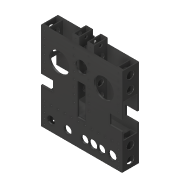
# Autodesk Inventor part: Kermit Elbow
Saved by Autodesk Inventor 2018.2 (Build 222227000, 227)
## iProperties
Created: 2018-02-12
Part Number: Kermit Elbow
Material: Glass
Document SubType Name: Modeling
Designer: lopez.xavier
Density: 2.18 g/cm^3
Appearance: Dark Gray
Author: lopez.xavier
Autodesk Inventor part; units mm, degrees
ref_plane "YZ Plane" through (0, 0, 0) normal (1, 0, 0) x (0, 1, 0)
ref_plane "XZ Plane" through (0, 0, 0) normal (0, 1, 0) x (-1, 0, 0)
ref_plane "XY Plane" through (0, 0, 0) normal (0, 0, 1) x (1, 0, 0)
sketch "Sketch1" plane through (0, 0, 0) normal (0, 0, 1) x (1, 0, 0)
  line L0 (0, 0) -> (304.8, 0)
  line L1 (304.8, 0) -> (304.8, 330.2)
  line L2 (304.8, 330.2) -> (0, 330.2)
  line L3 (0, 330.2) -> (0, 0)
  line L4 (0, 171.45) -> (45.72, 171.45)
  line L5 (45.72, 171.45) -> (45.72, 133.35)
  line L6 (45.72, 133.35) -> (0, 133.35)
  line L7 (0, 133.35) -> (0, 171.45)
  line L8 (304.8, 171.45) -> (259.08, 171.45)
  line L9 (259.08, 171.45) -> (259.08, 133.35)
  line L10 (259.08, 133.35) -> (304.8, 133.35)
  line L11 (304.8, 133.35) -> (304.8, 171.45)
  circle A0 centre (12.7, 317.5) radius 2.54
  circle A1 centre (292.1, 317.5) radius 2.54
  circle A2 centre (12.7, 292.1) radius 2.54
  circle A3 centre (12.7, 266.7) radius 2.54
  circle A4 centre (12.7, 241.3) radius 2.54
  circle A5 centre (12.7, 215.9) radius 2.54
  circle A6 centre (12.7, 190.5) radius 2.54
  circle A7 centre (292.1, 292.1) radius 2.54
  circle A8 centre (292.1, 266.7) radius 2.54
  circle A9 centre (292.1, 241.3) radius 2.54
  circle A10 centre (292.1, 215.9) radius 2.54
  circle A11 centre (292.1, 190.5) radius 2.54
  dimension "d0" = 304.8
  dimension "d1" = 330.2
  dimension "d2" = 158.75
  dimension "d3" = 38.1
  dimension "d4" = 45.72
  dimension "d5" = 45.72
  dimension "d6" = 5.08
  dimension "d7" = 5.08
  dimension "d8" = 12.7
  dimension "d9" = 12.7
  dimension "d10" = 12.7
  dimension "d11" = 12.7
  dimension "d14" = 25.4
  dimension "d21" = 25.4
  constraints: 24 end point, 12 centre point, 6 parallel, 4 point on line, 3 horizontal, 3 perpendicular, 2 vertical, 20 other
  measures "d0" distance of L0.start L0.end
  measures "d1" distance of L2.end L0.start
  measures "d2" distance between parallel lines of L2 L8
  measures "d3" distance between parallel lines of L4 L6
  measures "d4" distance between parallel lines of L3 L5
  measures "d5" distance between parallel lines of L1 L9
  measures "d6" diameter of A0
  measures "d7" diameter of A1
  measures "d8" distance from line of L2 A1.centre
  measures "d9" distance from line of L1 A1.centre
  measures "d10" distance from line of L2 A0.centre
  measures "d11" distance from line of L3 A0.centre
  measures "d14" distance of A0.centre A2.centre
  measures "d21" distance of A1.centre A7.centre
sketch "Sketch1 outline for Extrusion1" plane through (0, 0, 0) normal (0, 0, 1) x (1, 0, 0)
  line L0 (0, 330.2) -> (0, 171.45)
  line L1 (304.8, 330.2) -> (0, 330.2)
  line L2 (304.8, 171.45) -> (304.8, 330.2)
  line L3 (304.8, 171.45) -> (259.08, 171.45)
  line L4 (259.08, 171.45) -> (259.08, 133.35)
  line L5 (259.08, 133.35) -> (304.8, 133.35)
  line L6 (304.8, 0) -> (304.8, 133.35)
  line L7 (0, 0) -> (304.8, 0)
  line L8 (0, 133.35) -> (0, 0)
  line L9 (0, 133.35) -> (45.72, 133.35)
  line L10 (45.72, 133.35) -> (45.72, 171.45)
  line L11 (45.72, 171.45) -> (0, 171.45)
  circle A0 centre (12.7, 190.5) radius 2.54
  circle A1 centre (12.7, 215.9) radius 2.54
  circle A2 centre (12.7, 241.3) radius 2.54
  circle A3 centre (292.1, 190.5) radius 2.54
  circle A4 centre (292.1, 215.9) radius 2.54
  circle A5 centre (292.1, 241.3) radius 2.54
  circle A6 centre (12.7, 266.7) radius 2.54
  circle A7 centre (12.7, 292.1) radius 2.54
  circle A8 centre (12.7, 317.5) radius 2.54
  circle A9 centre (292.1, 266.7) radius 2.54
  circle A10 centre (292.1, 292.1) radius 2.54
  circle A11 centre (292.1, 317.5) radius 2.54
extrude "Extrusion1" add sketch "Sketch1 outline for Extrusion1" along normal blind 63.5
sketch "Sketch2" plane through (304.8, 171.45, 0) normal (1, 0, 0) x (0, 0, -1)
  line L0 (0, 158.75) -> (-63.5, 158.75) projected
  line L1 (0, -171.45) -> (-63.5, -171.45) projected
  line L2 (-57.531, 158.75) -> (-5.969, 158.75)
  line L3 (-5.969, 158.75) -> (-5.969, -171.45)
  line L4 (-5.969, -171.45) -> (-57.531, -171.45)
  line L5 (-57.531, -171.45) -> (-57.531, 158.75)
  line L6 (0, 0) -> (0, 158.75) projected
  line L7 (-63.5, 0) -> (-63.5, 158.75) projected
  dimension "d28" = 5.969
  dimension "d29" = 5.969
  constraints: 8 end point, 2 parallel, 2 point on line, 1 horizontal, 1 perpendicular
  measures "d28" distance between parallel lines of L6 L3
  measures "d29" distance between parallel lines of L7 L5
sketch "Sketch2 outline for Extrusion2" plane through (304.8, 171.45, 0) normal (1, 0, 0) x (0, 0, -1)
  line L0 (-57.531, 158.75) -> (-5.969, 158.75)
  line L1 (-5.969, 158.75) -> (-5.969, -171.45)
  line L2 (-5.969, -171.45) -> (-57.531, -171.45)
  line L3 (-57.531, -171.45) -> (-57.531, 158.75)
extrude "Extrusion2" cut sketch "Sketch2 outline for Extrusion2" against normal blind 508
sketch "Sketch3" plane through (0, 0, 63.5) normal (0, 0, 1) x (1, 0, 0)
  circle A0 centre (124.46, 317.5) radius 2.54
  line L0 (304.8, 330.2) -> (0, 330.2) projected
  line L1 (0, 330.2) -> (0, 171.45) projected
  circle A1 centre (124.46, 292.1) radius 2.54
  circle A2 centre (124.46, 266.7) radius 2.54
  circle A3 centre (124.46, 241.3) radius 2.54
  circle A4 centre (124.46, 215.9) radius 2.54
  circle A5 centre (124.46, 190.5) radius 2.54
  circle A6 centre (124.46, 165.1) radius 2.54
  circle A7 centre (124.46, 139.7) radius 2.54
  circle A8 centre (180.34, 317.5) radius 2.54
  circle A9 centre (180.34, 292.1) radius 2.54
  circle A10 centre (180.34, 266.7) radius 2.54
  circle A11 centre (180.34, 241.3) radius 2.54
  circle A12 centre (180.34, 215.9) radius 2.54
  circle A13 centre (180.34, 190.5) radius 2.54
  circle A14 centre (180.34, 165.1) radius 2.54
  circle A15 centre (180.34, 139.7) radius 2.54
  point P0 (0, 0)
  dimension "d32" = 5.08
  dimension "d33" = 12.7
  dimension "d34" = 124.46
  dimension "d37" = 25.4
  dimension "d40" = 55.88
  constraints: 16 centre point, 1 horizontal, 1 vertical, 30 other
  measures "d32" diameter of A0
  measures "d33" distance from line of L0 A0.centre
  measures "d34" distance from line of L1 A0.centre
  measures "d37" distance of A0.centre A1.centre
  measures "d40" distance of A0.centre A8.centre
sketch "Sketch3 outline for Extrusion3" plane through (0, 0, 63.5) normal (0, 0, 1) x (1, 0, 0)
  circle A0 centre (124.46, 317.5) radius 2.54
  circle A1 centre (124.46, 292.1) radius 2.54
  circle A2 centre (124.46, 266.7) radius 2.54
  circle A3 centre (124.46, 241.3) radius 2.54
  circle A4 centre (124.46, 215.9) radius 2.54
  circle A5 centre (124.46, 190.5) radius 2.54
  circle A6 centre (124.46, 165.1) radius 2.54
  circle A7 centre (124.46, 139.7) radius 2.54
  circle A8 centre (180.34, 317.5) radius 2.54
  circle A9 centre (180.34, 292.1) radius 2.54
  circle A10 centre (180.34, 266.7) radius 2.54
  circle A11 centre (180.34, 241.3) radius 2.54
  circle A12 centre (180.34, 215.9) radius 2.54
  circle A13 centre (180.34, 190.5) radius 2.54
  circle A14 centre (180.34, 165.1) radius 2.54
  circle A15 centre (180.34, 139.7) radius 2.54
extrude "Extrusion3" cut sketch "Sketch3 outline for Extrusion3" against normal blind 508
sketch "Sketch4" plane through (0, 0, 63.5) normal (0, 0, 1) x (1, 0, 0)
  line L0 (137.16, 216.662) -> (167.64, 216.662)
  line L1 (167.64, 216.662) -> (167.64, 97.282)
  line L2 (167.64, 97.282) -> (137.16, 97.282)
  line L3 (137.16, 97.282) -> (137.16, 216.662)
  circle A0 centre (124.46, 215.9) radius 2.54 projected
  line L4 (304.8, 330.2) -> (0, 330.2) projected
  point P0 (0, 0)
  dimension "d45" = 30.48
  dimension "d46" = 12.7
  dimension "d47" = 113.538
  dimension "d48" = 119.38
  constraints: 8 end point, 2 parallel, 1 horizontal, 1 perpendicular
  measures "d45" distance between parallel lines of L3 L1
  measures "d46" distance from line of A0.centre L3
  measures "d47" distance between parallel lines of L4 L0
  measures "d48" distance between parallel lines of L0 L2
sketch "Sketch4 outline for Extrusion4" plane through (0, 0, 63.5) normal (0, 0, 1) x (1, 0, 0)
  line L0 (137.16, 216.662) -> (167.64, 216.662)
  line L1 (167.64, 216.662) -> (167.64, 97.282)
  line L2 (167.64, 97.282) -> (137.16, 97.282)
  line L3 (137.16, 97.282) -> (137.16, 216.662)
extrude "Extrusion4" cut sketch "Sketch4 outline for Extrusion4" against normal blind 508
sketch "Sketch5" plane through (304.8, 171.45, 57.531) normal (0, 0, -1) x (-1, 0, 0)
  line L0 (304.8, 0) -> (304.8, 158.75) projected
  line L1 (304.8, 158.75) -> (279.4, 158.75)
  line L2 (279.4, 158.75) -> (279.4, 57.15)
  line L3 (279.4, 57.15) -> (304.8, 57.15)
  line L4 (304.8, 57.15) -> (304.8, 158.75)
  line L5 (0, 158.75) -> (0, 0) projected
  line L6 (0, 158.75) -> (25.4, 158.75)
  line L7 (25.4, 158.75) -> (25.4, 57.15)
  line L8 (25.4, 57.15) -> (0, 57.15)
  line L9 (0, 57.15) -> (0, 158.75)
  point P0 (304.8, -171.45)
  dimension "d51" = 25.4
  dimension "d52" = 101.6
  dimension "d53" = 25.4
  dimension "d54" = 101.6
  constraints: 16 end point, 4 parallel, 2 horizontal, 2 perpendicular
  measures "d51" distance of L3.end L2.end
  measures "d52" distance of L2.end L1.end
  measures "d53" distance of L7.end L8.end
  measures "d54" distance of L6.end L7.end
sketch "Sketch5 outline for Extrusion5" plane through (304.8, 171.45, 57.531) normal (0, 0, -1) x (-1, 0, 0)
  line L0 (304.8, 57.15) -> (304.8, 158.75)
  line L1 (279.4, 57.15) -> (304.8, 57.15)
  line L2 (279.4, 158.75) -> (279.4, 57.15)
  line L3 (304.8, 158.75) -> (279.4, 158.75)
  line L4 (0, 158.75) -> (25.4, 158.75)
  line L5 (25.4, 158.75) -> (25.4, 57.15)
  line L6 (25.4, 57.15) -> (0, 57.15)
  line L7 (0, 57.15) -> (0, 158.75)
extrude "Extrusion5" add sketch "Sketch5 outline for Extrusion5" along normal blind 51.562
sketch "Sketch6" plane through (0, 0, 63.5) normal (0, 0, 1) x (1, 0, 0)
  circle A0 centre (292.1, 241.3) radius 2.54 projected
  circle A1 centre (292.1, 266.7) radius 2.54 projected
  circle A2 centre (292.1, 292.1) radius 2.54 projected
  circle A3 centre (292.1, 317.5) radius 2.54 projected
  circle A4 centre (12.7, 317.5) radius 2.54 projected
  circle A5 centre (12.7, 292.1) radius 2.54 projected
  circle A6 centre (12.7, 266.7) radius 2.54 projected
  circle A7 centre (12.7, 241.3) radius 2.54 projected
  point P0 (0, 0)
sketch "Sketch6 outline for Extrusion6" plane through (0, 0, 63.5) normal (0, 0, 1) x (1, 0, 0)
  circle A0 centre (292.1, 241.3) radius 2.54
  circle A1 centre (292.1, 266.7) radius 2.54
  circle A2 centre (292.1, 292.1) radius 2.54
  circle A3 centre (292.1, 317.5) radius 2.54
  circle A4 centre (12.7, 317.5) radius 2.54
  circle A5 centre (12.7, 292.1) radius 2.54
  circle A6 centre (12.7, 266.7) radius 2.54
  circle A7 centre (12.7, 241.3) radius 2.54
extrude "Extrusion6" cut sketch "Sketch6 outline for Extrusion6" against normal blind 63.5
sketch "Sketch7" plane through (0, 0, 63.5) normal (0, 0, 1) x (1, 0, 0)
  circle A0 centre (68.58, 241.3) radius 38.1
  circle A1 centre (236.22, 241.3) radius 38.1
  circle A2 centre (12.7, 266.7) radius 2.54 projected
  circle A3 centre (292.1, 241.3) radius 2.54 projected
  line L0 (304.8, 330.2) -> (0, 330.2) projected
  point P0 (0, 0)
  dimension "d59" = 76.2
  dimension "d60" = 76.2
  dimension "d61" = 55.88
  dimension "d62" = 55.88
  dimension "d63" = 88.9
  dimension "d64" = 88.9
  constraints: 2 centre point
  measures "d59" diameter of A0
  measures "d60" diameter of A1
  measures "d61" horizontal distance of A2.centre A0.centre
  measures "d62" distance of A3.centre A1.centre
  measures "d63" distance from line of L0 A0.centre
  measures "d64" distance from line of L0 A1.centre
sketch "Sketch7 outline for Extrusion7" plane through (0, 0, 63.5) normal (0, 0, 1) x (1, 0, 0)
  circle A0 centre (68.58, 241.3) radius 38.1
  circle A1 centre (236.22, 241.3) radius 38.1
extrude "Extrusion7" cut sketch "Sketch7 outline for Extrusion7" against normal blind 63.5
sketch "Sketch8" plane through (304.8, 0, 57.531) normal (0, 0, -1) x (-1, 0, 0)
  line L0 (111.76, 152.4) -> (137.16, 152.4)
  line L1 (137.16, 152.4) -> (137.16, 355.6)
  line L2 (137.16, 355.6) -> (111.76, 355.6)
  line L3 (111.76, 355.6) -> (111.76, 152.4)
  line L4 (0, 330.2) -> (304.8, 330.2) projected
  circle A0 centre (124.46, 241.3) radius 2.54 projected
  line L5 (193.04, 152.4) -> (167.64, 152.4)
  line L6 (167.64, 152.4) -> (167.64, 355.6)
  line L7 (167.64, 355.6) -> (193.04, 355.6)
  line L8 (193.04, 355.6) -> (193.04, 152.4)
  circle A1 centre (180.34, 241.3) radius 2.54 projected
  point P0 (304.8, 0)
  dimension "d67" = 25.4
  dimension "d68" = 203.2
  dimension "d69" = 25.4
  dimension "d70" = 12.7
  dimension "d71" = 203.2
  dimension "d72" = 25.4
  dimension "d73" = 25.4
  dimension "d74" = 12.7
  constraints: 16 end point, 4 parallel, 2 horizontal, 2 perpendicular
  measures "d67" distance of L2.end L1.end
  measures "d68" distance of L1.end L0.end
  measures "d69" distance between parallel lines of L4 L2
  measures "d70" distance from line of A0.centre L3
  measures "d71" distance between parallel lines of L7 L5
  measures "d72" distance between parallel lines of L6 L8
  measures "d73" distance between parallel lines of L4 L7
  measures "d74" distance from line of A1.centre L8
sketch "Sketch8 outline for Extrusion8" plane through (304.8, 0, 57.531) normal (0, 0, -1) x (-1, 0, 0)
  line L0 (111.76, 355.6) -> (111.76, 152.4)
  line L1 (137.16, 355.6) -> (111.76, 355.6)
  line L2 (111.76, 152.4) -> (137.16, 152.4)
  line L3 (137.16, 152.4) -> (137.16, 355.6)
  circle A0 centre (124.46, 241.3) radius 2.54
  line L4 (193.04, 152.4) -> (167.64, 152.4)
  line L5 (193.04, 355.6) -> (193.04, 152.4)
  line L6 (167.64, 152.4) -> (167.64, 355.6)
  line L7 (167.64, 355.6) -> (193.04, 355.6)
  circle A1 centre (180.34, 241.3) radius 2.54
extrude "Extrusion8" add sketch "Sketch8 outline for Extrusion8" along normal blind 51.562
sketch "Sketch9" plane through (0, 0, 0) normal (0, 0, -1) x (-1, 0, 0)
  circle A0 centre (-180.34, 342.9) radius 2.54
  line L0 (-193.04, 355.6) -> (-193.04, 330.2) projected
  line L1 (-167.64, 355.6) -> (-193.04, 355.6) projected
  circle A1 centre (-180.34, 317.5) radius 2.54
  circle A2 centre (-180.34, 292.1) radius 2.54
  circle A3 centre (-180.34, 266.7) radius 2.54
  circle A4 centre (-180.34, 241.3) radius 2.54
  circle A5 centre (-180.34, 215.9) radius 2.54
  circle A6 centre (-180.34, 190.5) radius 2.54
  circle A7 centre (-180.34, 165.1) radius 2.54
  circle A8 centre (-124.46, 342.9) radius 2.54
  circle A9 centre (-124.46, 317.5) radius 2.54
  circle A10 centre (-124.46, 292.1) radius 2.54
  circle A11 centre (-124.46, 266.7) radius 2.54
  circle A12 centre (-124.46, 241.3) radius 2.54
  circle A13 centre (-124.46, 215.9) radius 2.54
  circle A14 centre (-124.46, 190.5) radius 2.54
  circle A15 centre (-124.46, 165.1) radius 2.54
  point P0 (0, 0)
  dimension "d77" = 5.08
  dimension "d78" = 12.7
  dimension "d79" = 12.7
  dimension "d82" = 25.4
  dimension "d85" = 55.88
  constraints: 16 centre point, 1 horizontal, 1 vertical, 30 other
  measures "d77" diameter of A0
  measures "d78" distance from line of L0 A0.centre
  measures "d79" distance from line of L1 A0.centre
  measures "d82" distance of A0.centre A1.centre
  measures "d85" distance of A0.centre A8.centre
sketch "Sketch9 outline for Extrusion9" plane through (0, 0, 0) normal (0, 0, -1) x (-1, 0, 0)
  circle A0 centre (-180.34, 342.9) radius 2.54
  circle A1 centre (-180.34, 317.5) radius 2.54
  circle A2 centre (-180.34, 292.1) radius 2.54
  circle A3 centre (-180.34, 266.7) radius 2.54
  circle A4 centre (-180.34, 241.3) radius 2.54
  circle A5 centre (-180.34, 215.9) radius 2.54
  circle A6 centre (-180.34, 190.5) radius 2.54
  circle A7 centre (-180.34, 165.1) radius 2.54
  circle A8 centre (-124.46, 342.9) radius 2.54
  circle A9 centre (-124.46, 317.5) radius 2.54
  circle A10 centre (-124.46, 292.1) radius 2.54
  circle A11 centre (-124.46, 266.7) radius 2.54
  circle A12 centre (-124.46, 241.3) radius 2.54
  circle A13 centre (-124.46, 215.9) radius 2.54
  circle A14 centre (-124.46, 190.5) radius 2.54
  circle A15 centre (-124.46, 165.1) radius 2.54
extrude "Extrusion9" cut sketch "Sketch9 outline for Extrusion9" against normal blind 63.5
sketch "Sketch10" plane through (304.8, 0, 57.531) normal (0, 0, -1) x (-1, 0, 0)
  line L0 (304.8, 0) -> (0, 0) projected
  line L1 (0, 0) -> (25.4, 0)
  line L2 (25.4, 0) -> (25.4, 101.6)
  line L3 (25.4, 101.6) -> (0, 101.6)
  line L4 (0, 101.6) -> (0, 0)
  line L5 (304.8, 0) -> (279.4, 0)
  line L6 (279.4, 0) -> (279.4, 101.6)
  line L7 (279.4, 101.6) -> (304.8, 101.6)
  line L8 (304.8, 101.6) -> (304.8, 0)
  dimension "d90" = 25.4
  dimension "d91" = 101.6
  dimension "d92" = 25.4
  dimension "d93" = 101.6
  constraints: 16 end point, 4 parallel, 2 horizontal, 2 perpendicular
  measures "d90" distance of L3.end L2.end
  measures "d91" distance of L2.end L1.end
  measures "d92" distance of L6.end L7.end
  measures "d93" distance of L5.end L6.end
sketch "Sketch10 outline for Extrusion10" plane through (304.8, 0, 57.531) normal (0, 0, -1) x (-1, 0, 0)
  line L0 (0, 101.6) -> (0, 0)
  line L1 (25.4, 101.6) -> (0, 101.6)
  line L2 (25.4, 0) -> (25.4, 101.6)
  line L3 (0, 0) -> (25.4, 0)
  line L4 (279.4, 0) -> (304.8, 0)
  line L5 (279.4, 101.6) -> (279.4, 0)
  line L6 (304.8, 101.6) -> (279.4, 101.6)
  line L7 (304.8, 0) -> (304.8, 101.6)
extrude "Extrusion10" add sketch "Sketch10 outline for Extrusion10" along normal blind 51.562
sketch "Sketch11" plane through (111.76, 355.6, 57.531) normal (0, 1, 0) x (1, 0, 0)
  line L0 (3.175, 3.175) -> (22.225, 3.175)
  line L1 (22.225, 3.175) -> (22.225, 48.387)
  line L2 (22.225, 48.387) -> (3.175, 48.387)
  line L3 (3.175, 48.387) -> (3.175, 3.175)
  line L4 (59.055, 3.175) -> (78.105, 3.175)
  line L5 (78.105, 3.175) -> (78.105, 48.387)
  line L6 (78.105, 48.387) -> (59.055, 48.387)
  line L7 (59.055, 48.387) -> (59.055, 3.175)
  line L8 (0, 0) -> (0, 51.562) projected
  line L9 (25.4, 0) -> (0, 0) projected
  line L10 (25.4, 0) -> (25.4, 51.562) projected
  line L11 (0, 51.562) -> (25.4, 51.562) projected
  line L12 (55.88, 0) -> (55.88, 51.562) projected
  line L13 (55.88, 0) -> (81.28, 0) projected
  line L14 (81.28, 0) -> (81.28, 51.562) projected
  line L15 (55.88, 51.562) -> (81.28, 51.562) projected
  line L16 (-89.535, 3.175) -> (-108.585, 3.175)
  line L17 (-108.585, 3.175) -> (-108.585, 48.387)
  line L18 (-108.585, 48.387) -> (-89.535, 48.387)
  line L19 (-89.535, 48.387) -> (-89.535, 3.175)
  line L20 (189.865, 48.387) -> (170.815, 48.387)
  line L21 (170.815, 48.387) -> (170.815, 3.175)
  line L22 (170.815, 3.175) -> (189.865, 3.175)
  line L23 (189.865, 3.175) -> (189.865, 48.387)
  line L24 (167.64, 0) -> (81.28, 0) projected
  line L25 (81.28, 51.562) -> (167.64, 51.562) projected
  line L26 (167.64, 0) -> (167.64, 51.562) projected
  line L27 (193.04, 57.531) -> (193.04, -5.969) projected
  line L28 (-111.76, 57.531) -> (-111.76, -5.969) projected
  line L29 (-86.36, 0) -> (-86.36, 51.562) projected
  line L30 (-86.36, 51.562) -> (0, 51.562) projected
  dimension "d96" = 3.175
  dimension "d97" = 3.175
  dimension "d98" = 3.175
  dimension "d99" = 3.175
  dimension "d100" = 3.175
  dimension "d101" = 3.175
  dimension "d102" = 3.175
  dimension "d103" = 3.175
  dimension "d104" = 3.175
  dimension "d105" = 3.175
  dimension "d106" = 3.175
  dimension "d107" = 3.175
  dimension "d108" = 3.175
  dimension "d109" = 3.175
  dimension "d110" = 3.175
  constraints: 32 end point, 8 parallel, 4 horizontal, 4 perpendicular, 1 point on line
  measures "d96" distance between parallel lines of L8 L3
  measures "d97" distance between parallel lines of L9 L0
  measures "d98" distance between parallel lines of L10 L1
  measures "d99" distance between parallel lines of L11 L2
  measures "d100" distance between parallel lines of L12 L7
  measures "d101" distance between parallel lines of L13 L4
  measures "d102" distance between parallel lines of L14 L5
  measures "d103" distance between parallel lines of L15 L6
  measures "d104" distance between parallel lines of L24 L22
  measures "d105" distance between parallel lines of L25 L20
  measures "d106" distance between parallel lines of L26 L21
  measures "d107" distance between parallel lines of L27 L23
  measures "d108" distance between parallel lines of L28 L17
  measures "d109" distance between parallel lines of L29 L19
  measures "d110" distance between parallel lines of L30 L18
sketch "Sketch11 outline for Extrusion11" plane through (111.76, 355.6, 57.531) normal (0, 1, 0) x (1, 0, 0)
  line L0 (-89.535, 3.175) -> (-108.585, 3.175)
  line L1 (-108.585, 3.175) -> (-108.585, 48.387)
  line L2 (-108.585, 48.387) -> (-89.535, 48.387)
  line L3 (-89.535, 48.387) -> (-89.535, 3.175)
  line L4 (189.865, 3.175) -> (189.865, 48.387)
  line L5 (170.815, 3.175) -> (189.865, 3.175)
  line L6 (170.815, 48.387) -> (170.815, 3.175)
  line L7 (189.865, 48.387) -> (170.815, 48.387)
  line L8 (3.175, 48.387) -> (3.175, 3.175)
  line L9 (22.225, 48.387) -> (3.175, 48.387)
  line L10 (22.225, 3.175) -> (22.225, 48.387)
  line L11 (3.175, 3.175) -> (22.225, 3.175)
  line L12 (59.055, 48.387) -> (59.055, 3.175)
  line L13 (78.105, 48.387) -> (59.055, 48.387)
  line L14 (78.105, 3.175) -> (78.105, 48.387)
  line L15 (59.055, 3.175) -> (78.105, 3.175)
extrude "Extrusion11" cut sketch "Sketch11 outline for Extrusion11" against normal blind 381
sketch "Sketch12" plane through (304.8, 0, 0) normal (1, 0, 0) x (0, 0, -1)
  circle A0 centre (-31.75, 73.66) radius 13.97
  line L0 (-57.531, 101.6) -> (-5.969, 101.6) projected
  line L1 (-63.5, 0) -> (-63.5, 133.35) projected
  circle A1 centre (-31.75, 25.4) radius 13.97
  point P0 (0, 0)
  dimension "d113" = 27.94
  dimension "d125" = 27.94
  dimension "d126" = 31.75
  dimension "d127" = 27.94
  dimension "d128" = 31.75
  dimension "d129" = 48.26
  constraints: 2 centre point
  measures "d113" diameter of A0
  measures "d125" distance from line of L0 A0.centre
  measures "d126" distance from line of L1 A0.centre
  measures "d127" diameter of A1
  measures "d128" distance from line of L1 A1.centre
  measures "d129" distance of A0.centre A1.centre
sketch "Sketch13" plane through (25.4, 0, 57.531) normal (1, 0, 0) x (0, 0, -1)
  line L0 (0, 0) -> (0, 101.6) projected
  line L1 (0, 99.06) -> (51.562, 99.06)
  line L2 (51.562, 99.06) -> (51.562, 73.66)
  line L3 (51.562, 73.66) -> (0, 73.66)
  line L4 (0, 73.66) -> (0, 99.06)
  line L5 (0, 101.6) -> (51.562, 101.6) projected
  point P0 (57.531, 0)
  dimension "d114" = 51.562
  dimension "d115" = 25.4
  dimension "d116" = 2.54
  constraints: 8 end point, 2 parallel, 1 horizontal, 1 perpendicular, 1 point on line
  measures "d114" distance of L2.end L3.end
  measures "d115" distance of L1.end L2.end
  measures "d116" distance between parallel lines of L5 L1
sketch "Sketch13 outline for Extrusion12" plane through (25.4, 0, 57.531) normal (1, 0, 0) x (0, 0, -1)
  line L0 (0, 99.06) -> (51.562, 99.06)
  line L1 (51.562, 99.06) -> (51.562, 73.66)
  line L2 (51.562, 73.66) -> (0, 73.66)
  line L3 (0, 73.66) -> (0, 99.06)
extrude "Extrusion12" add sketch "Sketch13 outline for Extrusion12" along normal blind 254
sketch "Sketch14" plane through (279.4, 0, 5.969) normal (-1, 0, 0) x (0, 0, 1)
  line L0 (3.175, 76.835) -> (48.387, 76.835)
  line L1 (48.387, 76.835) -> (48.387, 95.885)
  line L2 (48.387, 95.885) -> (3.175, 95.885)
  line L3 (3.175, 95.885) -> (3.175, 76.835)
  line L4 (0, 73.66) -> (51.562, 73.66) projected
  line L5 (51.562, 99.06) -> (0, 99.06) projected
  line L6 (0, 97.282) -> (0, 99.06) projected
  line L7 (48.387, 101.6) -> (48.387, 0) projected
  point P0 (-5.969, 0)
  dimension "d119" = 3.175
  dimension "d120" = 3.175
  dimension "d121" = 3.175
  dimension "d122" = 0
  constraints: 8 end point, 2 parallel, 1 horizontal, 1 perpendicular
  measures "d119" distance between parallel lines of L4 L0
  measures "d120" distance between parallel lines of L5 L2
  measures "d121" distance between parallel lines of L6 L3
  measures "d122" distance between parallel lines of L7 L1
sketch "Sketch14 outline for Extrusion13" plane through (279.4, 0, 5.969) normal (-1, 0, 0) x (0, 0, 1)
  line L0 (3.175, 95.885) -> (3.175, 76.835)
  line L1 (48.387, 95.885) -> (3.175, 95.885)
  line L2 (48.387, 76.835) -> (48.387, 95.885)
  line L3 (3.175, 76.835) -> (48.387, 76.835)
extrude "Extrusion13" cut sketch "Sketch14 outline for Extrusion13" along normal blind 254
sketch "Sketch12 outline for Extrusion14" plane through (304.8, 0, 0) normal (1, 0, 0) x (0, 0, -1)
  circle A0 centre (-31.75, 73.66) radius 13.97
  circle A1 centre (-31.75, 25.4) radius 13.97
extrude "Extrusion14" cut sketch "Sketch12 outline for Extrusion14" against normal blind 25.4
sketch "Sketch15" plane through (0, 0, 0) normal (-1, 0, 0) x (0, 0, 1)
  circle A0 centre (31.75, 73.66) radius 13.97 projected
  circle A1 centre (31.75, 73.66) radius 13.97
  circle A2 centre (31.75, 25.4) radius 13.97 projected
  circle A3 centre (31.75, 25.4) radius 13.97
  point P0 (0, 0)
  constraints: 2 centre point, 2 coincident
sketch "Sketch15 outline for Extrusion15" plane through (0, 0, 0) normal (-1, 0, 0) x (0, 0, 1)
  circle A0 centre (31.75, 73.66) radius 13.97
  circle A1 centre (31.75, 25.4) radius 13.97
extrude "Extrusion15" cut sketch "Sketch15 outline for Extrusion15" against normal blind 25.4
sketch "Sketch16" plane through (304.8, 171.45, 0) normal (1, 0, 0) x (0, 0, -1)
  circle A0 centre (-31.75, 130.81) radius 13.97
  circle A1 centre (-31.75, 82.55) radius 13.97
  line L0 (0, 0) -> (0, 158.75) projected
  line L1 (0, 158.75) -> (-63.5, 158.75) projected
  point P0 (0, -171.45)
  dimension "d134" = 27.94
  dimension "d135" = 27.94
  dimension "d136" = 31.75
  dimension "d137" = 31.75
  dimension "d138" = 27.94
  dimension "d139" = 48.26
  constraints: 2 centre point
  measures "d134" diameter of A0
  measures "d135" diameter of A1
  measures "d136" distance from line of L0 A0.centre
  measures "d137" distance from line of L0 A1.centre
  measures "d138" distance from line of L1 A0.centre
  measures "d139" distance of A0.centre A1.centre
sketch "Sketch16 outline for Extrusion16" plane through (304.8, 171.45, 0) normal (1, 0, 0) x (0, 0, -1)
  circle A0 centre (-31.75, 130.81) radius 13.97
  circle A1 centre (-31.75, 82.55) radius 13.97
extrude "Extrusion16" cut sketch "Sketch16 outline for Extrusion16" against normal blind 25.4
sketch "Sketch17" plane through (0, 171.45, 0) normal (-1, 0, 0) x (0, 0, 1)
  circle A0 centre (31.75, 130.81) radius 13.97 projected
  circle A1 centre (31.75, 82.55) radius 13.97 projected
  circle A2 centre (31.75, 130.81) radius 13.97
  circle A3 centre (31.75, 82.55) radius 13.97
  point P0 (0, -171.45)
  constraints: 2 centre point, 2 coincident, 2 concentric
sketch "Sketch17 outline for Extrusion17" plane through (0, 171.45, 0) normal (-1, 0, 0) x (0, 0, 1)
  circle A0 centre (31.75, 130.81) radius 13.97
  circle A1 centre (31.75, 82.55) radius 13.97
extrude "Extrusion17" cut sketch "Sketch17 outline for Extrusion17" against normal blind 25.4
sketch "Sketch18" plane through (193.04, 330.2, 57.531) normal (1, 0, 0) x (0, 0, -1)
  circle A0 centre (25.781, -152.4) radius 11.43
  line L0 (0, -177.8) -> (51.562, -177.8) projected
  line L1 (0, -177.8) -> (0, 0) projected
  circle A1 centre (25.781, -107.95) radius 11.43
  circle A2 centre (25.781, -63.5) radius 11.43
  point P0 (57.531, -330.2)
  dimension "d152" = 25.4
  dimension "d144" = 22.86
  dimension "d145" = 25.4
  dimension "d146" = 25.781
  dimension "d149" = 44.45
  constraints: 3 centre point, 1 vertical, 4 other
  measures "d144" diameter of A0
  measures "d145" distance from line of L0 A0.centre
  measures "d146" distance from line of L1 A0.centre
  measures "d149" distance of A0.centre A1.centre
sketch "Sketch18 outline for Extrusion18" plane through (193.04, 330.2, 57.531) normal (1, 0, 0) x (0, 0, -1)
  circle A0 centre (25.781, -152.4) radius 11.43
  circle A1 centre (25.781, -107.95) radius 11.43
  circle A2 centre (25.781, -63.5) radius 11.43
extrude "Extrusion18" cut sketch "Sketch18 outline for Extrusion18" against normal blind 127
sketch "Sketch19" plane through (0, 0, 63.5) normal (0, 0, 1) x (1, 0, 0)
  circle A0 centre (267.97, 37.592) radius 15.875
  line L0 (304.8, 0) -> (304.8, 133.35) projected
  line L1 (0, 0) -> (304.8, 0) projected
  circle A1 centre (195.834, 37.592) radius 15.875
  circle A2 centre (37.338, 37.592) radius 14.224
  line L2 (0, 133.35) -> (0, 0) projected
  circle A3 centre (100.711, 37.592) radius 14.224
  circle A4 centre (164.084, 37.592) radius 14.224
  circle A5 centre (227.457, 37.592) radius 14.224
  dimension "d156" = 31.75
  dimension "d157" = 36.83
  dimension "d160" = 72.136
  dimension "d165" = 28.448
  dimension "d166" = 37.338
  dimension "d169" = 63.373
  dimension "d174" = 37.592
  dimension "d175" = 37.592
  constraints: 6 centre point, 2 horizontal, 8 other
  measures "d156" diameter of A0
  measures "d157" distance from line of L0 A0.centre
  measures "d160" distance of A0.centre A1.centre
  measures "d165" diameter of A2
  measures "d166" distance from line of L2 A2.centre
  measures "d169" distance of A2.centre A3.centre
  measures "d174" distance from line of L1 A0.centre
  measures "d175" distance from line of L1 A2.centre
sketch "Sketch19 outline for Extrusion19" plane through (0, 0, 63.5) normal (0, 0, 1) x (1, 0, 0)
  circle A0 centre (37.338, 37.592) radius 14.224
  circle A1 centre (100.711, 37.592) radius 14.224
  circle A2 centre (164.084, 37.592) radius 14.224
  circle A3 centre (227.457, 37.592) radius 14.224
  circle A4 centre (267.97, 37.592) radius 15.875
  circle A5 centre (195.834, 37.592) radius 15.875
extrude "Extrusion19" cut sketch "Sketch19 outline for Extrusion19" against normal blind 5.969
sketch "Sketch20" plane through (0, 0, 0) normal (0, 0, -1) x (-1, 0, 0)
  circle A0 centre (-254, 37.592) radius 14.224
  line L0 (0, 0) -> (-304.8, 0) projected
  line L1 (-304.8, 0) -> (-304.8, 133.35) projected
  circle A1 centre (-203.2, 37.592) radius 14.224
  circle A2 centre (-152.4, 37.592) radius 14.224
  circle A3 centre (-101.6, 37.592) radius 14.224
  circle A4 centre (-50.8, 37.592) radius 14.224
  dimension "d178" = 28.448
  dimension "d179" = 37.592
  dimension "d180" = 50.8
  dimension "d183" = 50.8
  constraints: 5 centre point, 1 horizontal, 8 other
  measures "d178" diameter of A0
  measures "d179" distance from line of L0 A0.centre
  measures "d180" distance from line of L1 A0.centre
  measures "d183" distance of A0.centre A1.centre
sketch "Sketch20 outline for Extrusion20" plane through (0, 0, 0) normal (0, 0, -1) x (-1, 0, 0)
  circle A0 centre (-254, 37.592) radius 14.224
  circle A1 centre (-203.2, 37.592) radius 14.224
  circle A2 centre (-152.4, 37.592) radius 14.224
  circle A3 centre (-101.6, 37.592) radius 14.224
  circle A4 centre (-50.8, 37.592) radius 14.224
extrude "Extrusion20" cut sketch "Sketch20 outline for Extrusion20" against normal blind 5.969
sketch "Sketch21" plane through (0, 0, 63.5) normal (0, 0, 1) x (1, 0, 0)
  circle A0 centre (152.4, 267.462) radius 22.86
  line L0 (137.16, 97.282) -> (137.16, 216.662) projected
  line L1 (137.16, 216.662) -> (167.64, 216.662) projected
  point P0 (0, 0)
  dimension "d190" = 45.72
  dimension "d191" = 15.24
  dimension "d192" = 50.8
  constraints: 1 centre point
  measures "d190" diameter of A0
  measures "d191" distance from line of A0.centre L0
  measures "d192" distance from line of A0.centre L1
sketch "Sketch21 outline for Extrusion21" plane through (0, 0, 63.5) normal (0, 0, 1) x (1, 0, 0)
  circle A0 centre (152.4, 267.462) radius 22.86
extrude "Extrusion21" cut sketch "Sketch21 outline for Extrusion21" against normal blind 5.969
sketch "Sketch22" plane through (0, 0, 63.5) normal (0, 0, 1) x (1, 0, 0)
  circle A0 centre (12.7, 12.7) radius 2.54
  line L0 (0, 133.35) -> (0, 0) projected
  line L1 (0, 0) -> (304.8, 0) projected
  circle A1 centre (12.7, 31.75) radius 2.54
  circle A2 centre (12.7, 50.8) radius 2.54
  circle A3 centre (12.7, 69.85) radius 2.54
  circle A4 centre (12.7, 88.9) radius 2.54
  circle A5 centre (292.1, 12.7) radius 2.54
  circle A6 centre (292.1, 31.75) radius 2.54
  circle A7 centre (292.1, 50.8) radius 2.54
  circle A8 centre (292.1, 69.85) radius 2.54
  circle A9 centre (292.1, 88.9) radius 2.54
  dimension "d195" = 5.08
  dimension "d196" = 12.7
  dimension "d197" = 12.7
  dimension "d200" = 19.05
  dimension "d203" = 279.4
  constraints: 10 centre point, 1 horizontal, 1 vertical, 18 other
  measures "d195" diameter of A0
  measures "d196" distance from line of L0 A0.centre
  measures "d197" distance from line of L1 A0.centre
  measures "d200" distance of A0.centre A1.centre
  measures "d203" distance of A0.centre A5.centre
sketch "Sketch22 outline for Extrusion22" plane through (0, 0, 63.5) normal (0, 0, 1) x (1, 0, 0)
  circle A0 centre (12.7, 12.7) radius 2.54
  circle A1 centre (12.7, 31.75) radius 2.54
  circle A2 centre (12.7, 50.8) radius 2.54
  circle A3 centre (12.7, 69.85) radius 2.54
  circle A4 centre (12.7, 88.9) radius 2.54
  circle A5 centre (292.1, 12.7) radius 2.54
  circle A6 centre (292.1, 31.75) radius 2.54
  circle A7 centre (292.1, 50.8) radius 2.54
  circle A8 centre (292.1, 69.85) radius 2.54
  circle A9 centre (292.1, 88.9) radius 2.54
extrude "Extrusion22" cut sketch "Sketch22 outline for Extrusion22" against normal blind 279.4
sketch "Sketch23" plane through (0, 0, 63.5) normal (0, 0, 1) x (1, 0, 0)
  circle A0 centre (38.735, 86.36) radius 2.54
  circle A1 centre (12.7, 69.85) radius 2.54 projected
  line L0 (0, 133.35) -> (0, 0) projected
  circle A2 centre (12.7, 88.9) radius 2.54 projected
  line L1 (0, 0) -> (304.8, 0) projected
  circle A3 centre (64.135, 86.36) radius 2.54
  circle A4 centre (89.535, 86.36) radius 2.54
  circle A5 centre (114.935, 86.36) radius 2.54
  circle A6 centre (140.335, 86.36) radius 2.54
  circle A7 centre (165.735, 86.36) radius 2.54
  circle A8 centre (191.135, 86.36) radius 2.54
  circle A9 centre (216.535, 86.36) radius 2.54
  circle A10 centre (241.935, 86.36) radius 2.54
  circle A11 centre (267.335, 86.36) radius 2.54
  line L2 (279.4, 76.835) -> (25.4, 76.835) projected
  dimension "d208" = 5.08
  dimension "d210" = 38.735
  dimension "d213" = 25.4
  dimension "d220" = 9.525
  constraints: 10 centre point, 1 horizontal, 18 other
  measures "d208" diameter of A0
  measures "d210" distance from line of L0 A0.centre
  measures "d213" distance of A0.centre A3.centre
  measures "d220" distance from line of A0.centre L2
sketch "Sketch23 outline for Extrusion23" plane through (0, 0, 63.5) normal (0, 0, 1) x (1, 0, 0)
  circle A0 centre (38.735, 86.36) radius 2.54
  circle A1 centre (64.135, 86.36) radius 2.54
  circle A2 centre (89.535, 86.36) radius 2.54
  circle A3 centre (114.935, 86.36) radius 2.54
  circle A4 centre (140.335, 86.36) radius 2.54
  circle A5 centre (165.735, 86.36) radius 2.54
  circle A6 centre (191.135, 86.36) radius 2.54
  circle A7 centre (216.535, 86.36) radius 2.54
  circle A8 centre (241.935, 86.36) radius 2.54
  circle A9 centre (267.335, 86.36) radius 2.54
extrude "Extrusion23" cut sketch "Sketch23 outline for Extrusion23" against normal blind 127
sketch "Sketch24" plane through (193.04, 330.2, 57.531) normal (1, 0, 0) x (0, 0, -1)
  circle A0 centre (25.781, 12.7) radius 6.35
  line L0 (0, 25.4) -> (51.562, 25.4) projected
  line L1 (51.562, 25.4) -> (51.562, 0) projected
  point P0 (57.531, -330.2)
  dimension "d223" = 12.7
  dimension "d224" = 12.7
  dimension "d225" = 25.781
  constraints: 1 centre point
  measures "d223" diameter of A0
  measures "d224" distance from line of L0 A0.centre
  measures "d225" distance from line of L1 A0.centre
sketch "Sketch25" plane through (0, 0, 0) normal (0, 0, -1) x (-1, 0, 0)
  line L0 (-137.16, 330.2) -> (-137.16, 216.662) projected
  line L1 (-167.64, 216.662) -> (-137.16, 216.662)
  line L2 (-137.16, 216.662) -> (-137.16, 330.2)
  line L3 (-137.16, 330.2) -> (-167.64, 330.2)
  line L4 (-167.64, 330.2) -> (-167.64, 216.662)
  point P0 (0, 0)
  constraints: 8 end point, 2 parallel, 1 horizontal, 1 perpendicular
sketch "Sketch25 outline for Extrusion24" plane through (0, 0, 0) normal (0, 0, -1) x (-1, 0, 0)
  line L0 (-167.64, 330.2) -> (-167.64, 216.662)
  line L1 (-137.16, 330.2) -> (-167.64, 330.2)
  line L2 (-137.16, 216.662) -> (-137.16, 330.2)
  line L3 (-167.64, 216.662) -> (-137.16, 216.662)
extrude "Extrusion24" cut sketch "Sketch25 outline for Extrusion24" against normal blind 5.969
sketch "Sketch24 outline for Extrusion25" plane through (193.04, 330.2, 57.531) normal (1, 0, 0) x (0, 0, -1)
  circle A0 centre (25.781, 12.7) radius 6.35
extrude "Extrusion25" cut sketch "Sketch24 outline for Extrusion25" against normal blind 101.6
sketch "Sketch26" plane through (304.8, 171.45, 0) normal (1, 0, 0) x (0, 0, -1)
  circle A0 centre (-31.75, 130.81) radius 13.97 projected
  point P0 (0, -171.45)
sketch "Sketch26 outline for Extrusion26" plane through (304.8, 171.45, 0) normal (1, 0, 0) x (0, 0, -1)
  circle A0 centre (-31.75, 130.81) radius 13.97
extrude "Extrusion26" cut sketch "Sketch26 outline for Extrusion26" against normal blind 381
equation "\"d5\" = d4"
equation "\"d10\" = d8"
equation "\"d11\" = d9"
equation "\"d29\" = d28"
equation "\"d62\" = d61"
equation "\"d64\" = d63"
equation "\"d67\" = d72"
equation "\"d68\" = d71"
equation "\"d127\" = d113"
equation "\"d128\" = d126"
equation "\"d120\" = d119"
equation "\"d121\" = d119"
equation "\"d135\" = d134"
equation "\"d137\" = d136"
equation "\"d175\" = d174"
equation "\"d206\" = d203"
body "Solid1"
